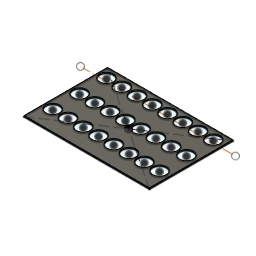
masque bcr2000 v5 (Autodesk Fusion 360 design; units mm, degrees)
Autodesk Fusion 360 part; units mm, degrees
sketch "Esquisse1" plane through (0, 0, 0) normal (0, 0, 1) x (1, 0, 0)
  line L0 (118, -78.5) -> (-118, -78.5)
  line L1 (-118, -78.5) -> (-118, 78.5)
  line L2 (-118, 78.5) -> (118, 78.5)
  line L3 (118, 78.5) -> (118, -78.5)
  line L4 (118, -78.5) -> (-118, 78.5) construction
  line L5 (-118, -78.5) -> (118, 78.5) construction
  circle A0 centre (-102, 60.5) radius 13
  line L6 (-147.0099, 56.5) -> (145.0532, 56.5) construction
  circle A1 centre (-73.25, 60.5) radius 13
  circle A2 centre (-44.5, 60.5) radius 13
  circle A3 centre (-15.75, 60.5) radius 13
  circle A4 centre (13, 60.5) radius 13
  circle A5 centre (41.75, 60.5) radius 13
  circle A6 centre (70.5, 60.5) radius 13
  circle A7 centre (99.25, 60.5) radius 13
  circle A8 centre (-102, 9.84) radius 13
  circle A9 centre (-73.25, 9.84) radius 13
  circle A10 centre (-44.5, 9.84) radius 13
  circle A11 centre (-15.75, 9.84) radius 13
  circle A12 centre (13, 9.84) radius 13
  circle A13 centre (41.75, 9.84) radius 13
  circle A14 centre (70.5, 9.84) radius 13
  circle A15 centre (99.25, 9.84) radius 13
  circle A16 centre (-102, -40.82) radius 13
  circle A17 centre (-73.25, -40.82) radius 13
  circle A18 centre (-44.5, -40.82) radius 13
  circle A19 centre (-15.75, -40.82) radius 13
  circle A20 centre (13, -40.82) radius 13
  circle A21 centre (41.75, -40.82) radius 13
  circle A22 centre (70.5, -40.82) radius 13
  circle A23 centre (99.25, -40.82) radius 13
  dimension "d1" = 236
  dimension "d2" = 157
  dimension "d3" = 26
  dimension "d4" = 18
  dimension "d5" = 16
  dimension "d9" = 28.75
  dimension "d10" = -50.66
  constraint horizontal L0
  constraint perpendicular L0 L1
  constraint parallel L0 L2
  constraint parallel L1 L3
  constraint coincident L4 origin
  constraint coincident L5 origin
  constraint horizontal L6
  measures "d1" distance of L1.end L2.end
  measures "d2" distance of L0.end L1.end
  measures "d3" diameter of A0
  measures "d4" distance of L2 A0.centre
  measures "d5" distance of L1 A0.centre
extrude "Extrusion1" add sketch "Esquisse1" along normal blind 2
